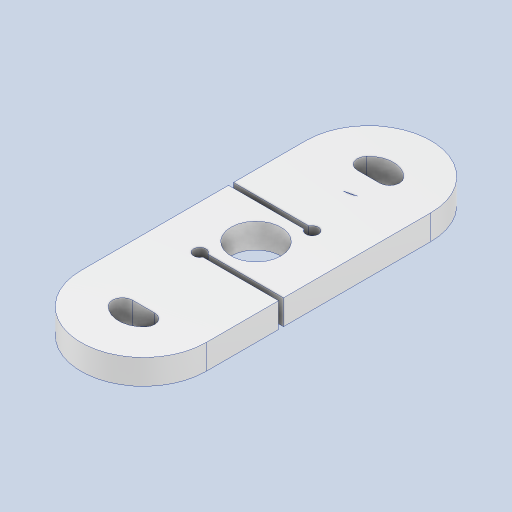
# Autodesk Inventor part: mod6
Saved by Autodesk Inventor 2024 (Build 280153000, 153)
## iProperties
Created: 2025-12-02
Part Number: mod6
Material: Aluminio 6061
Document SubType Name: Modeling
Designer: ANDRES
Density: 2.7 g/cm^3
Appearance: Aluminio - Plano
Author: ANDRES
Autodesk Inventor part; units mm, degrees
ref_plane "YZ Plane" through (0, 0, 0) normal (1, 0, 0) x (0, 1, 0)
ref_plane "XZ Plane" through (0, 0, 0) normal (0, 1, 0) x (-1, 0, 0)
ref_plane "XY Plane" through (0, 0, 0) normal (0, 0, 1) x (1, 0, 0)
sketch "Boceto1" plane through (0, 0, 0) normal (0, 1, 0) x (-1, 0, 0)
  circle A0 centre (0, -45) radius 10
  circle A1 centre (0, 45) radius 10
  line L0 (0.0371, -35.0001) -> (-0.0371, -35.0001)
  line L1 (0.0371, -35.0001) -> (-4.4959, -36.0676)
  circle A2 centre (0, -45) radius 25
  circle A3 centre (0, 45) radius 25
  line L2 (0, 89.4288) -> (0, -73.1924) construction
  line L3 (-38.8142, 0) -> (36.7218, 0) construction
  line L4 (0, 45) -> (0, -45)
  line L5 (10, 45) -> (-10, 45)
  line L6 (10, -45) -> (-10, -45)
  line L7 (25, 45) -> (25, -45)
  line L8 (-25, -45) -> (-25, 45)
  circle A4 centre (0, 0) radius 10
  circle A5 centre (7.5, 15) radius 2.5
  line L9 (-25, 14) -> (5.2087, 14)
  line L10 (5.2087, 14) -> (5.2087, 16)
  line L11 (5.2087, 16) -> (-25, 16)
  line L12 (-25, 16) -> (-25, 14)
  line L13 (-25, 14) -> (5.2087, 16) construction
  line L14 (5.2087, 14) -> (-25, 16) construction
  line L15 (10, 0) -> (10, 38.9395) construction
  circle A6 centre (-7.5, -15) radius 2.5
  line L16 (25, -16) -> (-5.2087, -16)
  line L17 (-5.2087, -16) -> (-5.2087, -14)
  line L18 (-5.2087, -14) -> (25, -14)
  line L19 (25, -14) -> (25, -16)
  line L20 (25, -16) -> (-5.2087, -14) construction
  line L21 (-5.2087, -16) -> (25, -14) construction
  line L22 (-10, 0) -> (-10, -29.6504) construction
  point P0 (0, 60)
  point P1 (0, -60)
  point P2 (-0.0332, 54.9999)
  point P3 (-0.0332, 54.9999)
  point P4 (-12.4808, 36.6795)
  point P5 (11.1803, 35)
  point P6 (-9.8956, 15)
  point P7 (-9.8956, 15)
  point P8 (-25, 15)
  point P9 (9.8956, -15)
  point P10 (9.8956, -15)
  point P11 (25, -15)
  point P12 (25, -16)
  point P13 (-5.2087, -16)
  point P14 (25, -14)
  point P15 (5.2087, 14)
  dimension "d48" = 5
  dimension "d51" = 5
  dimension "d42" = 50
  dimension "d43" = 50
  dimension "d44" = 90
  dimension "d45" = 20
  dimension "d46" = 20
  dimension "d47" = 20
  dimension "d49" = 2
  dimension "d50" = 14
  dimension "d52" = 2
  dimension "d53" = 14
  constraints: 46 end point, 15 point on circle, 9 midpoint, 6 tangent, 5 centre point, 5 parallel, 5 perpendicular, 5 point on line, 5 vertical, 4 horizontal, 3 coincident, 2 horizontal alignment, 2 vertical alignment, 1 concentric, 10 other
  measures "d42" diameter of A3
  measures "d43" diameter of A2
  measures "d44" distance of L4.start L4.end
  measures "d45" diameter of A1
  measures "d46" diameter of A0
  measures "d47" diameter of A4
  measures "d49" distance of L11.end L9.start
  measures "d50" distance from line of A4.centre L9
  measures "d52" distance of L18.end L16.start
  measures "d53" distance from line of A4.centre L18
extrude "Extrusión9" add sketch "Boceto1" along normal blind 10 contours L6 L4 L1 A0 | A0 L1 L4 L6 | A1 L4 L5 | L5 L4 A1 | A2 | L8 L9 L4 A4 L18 A6 L16 A2 | A2 L4 L16 L7 | L8 A3 L4 L11 | L9 A5 L11 L4 A3 L7 L18 A4 | A3
fillet "Empalme3" radius 4 4 edges at (-10, 5, -45) (10, 5, -45) (-10, 5, 45) (10, 5, 45)
